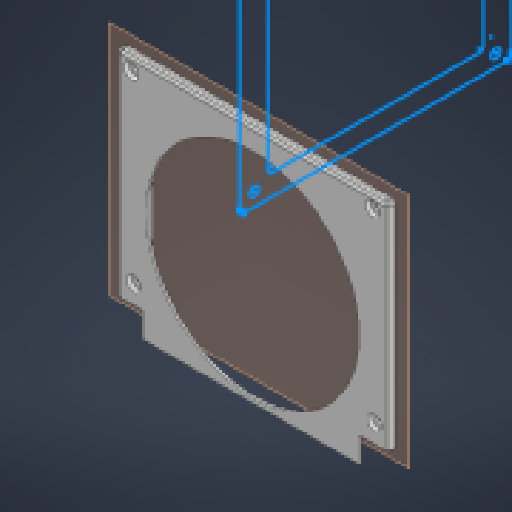
# Autodesk Inventor part: BP_FanCover
Saved by Autodesk Inventor 2026.1 (Build 301233020, 233B)
## iProperties
Created: 2025-09-13
Part Number: BP_FanCover
Material: Generic
Document SubType Name: Modeling
Designer: atrus
Density: 1 g/cm^3
Appearance: Default
Author: atrus
Autodesk Inventor part; units mm, degrees
ref_plane "YZ Plane" through (0, 0, 0) normal (1, 0, 0) x (0, 1, 0)
ref_plane "XZ Plane" through (0, 0, 0) normal (0, 1, 0) x (-1, 0, 0)
ref_plane "XY Plane" through (0, 0, 0) normal (0, 0, 1) x (1, 0, 0)
ref_plane "Work Plane1" through (0, 0, 0) normal (0, 0, 1) x (1, 0, 0)
sketch "Sketch1" plane through (0, 0, 0) normal (0, 0, 1) x (1, 0, 0)
  circle A0 centre (-100.824, -72) radius 2
  circle A1 centre (2.867, -72) radius 2
  circle A2 centre (-101.9061, 6.8071) radius 2
  circle A3 centre (2.0738, 7.3071) radius 2
  spline S0 degree 3 poles (-108.332, 10.6) (-108.332, 10.8603) (-108.2812, 11.1181) (-108.0835, 11.5997) (-107.9386, 11.819) (-107.5727, 12.1898) (-107.3552, 12.3377) (-106.9918, 12.4925) (-106.8631, 12.5326) (-106.5995, 12.5864) (-106.4653, 12.6) (-106.3308, 12.6) knots 0 0 0 0 0.247849 0.247849 0.495777 0.495777 0.743857 0.743857 0.871926 0.871926 1 1 1 1
  line L0 (-108.332, 10.6) -> (-108.332, -80)
  line L1 (-96.066, -80) -> (-108.332, -80)
  line L2 (-96.066, -80) -> (-96.066, 1.6)
  arc A4 (-94.066, 3.6) -> (-96.066, 1.6) centre (-94.066, 1.6) ccw
  line L3 (-94.066, 3.6) -> (-5.266, 3.6)
  arc A5 (-3.266, 1.6) -> (-5.266, 3.6) centre (-5.266, 1.6) ccw
  line L4 (-3.266, -80) -> (-3.266, 1.6)
  line L5 (-3.266, -80) -> (9, -80)
  line L6 (9, 10.6) -> (9, -80)
  spline S1 degree 3 poles (6.9988, 12.6) (7.2595, 12.6) (7.5178, 12.5491) (8.0001, 12.3511) (8.2196, 12.206) (8.5905, 11.8399) (8.7383, 11.6225) (8.8929, 11.2593) (8.9329, 11.1309) (8.9865, 10.868) (9, 10.7342) (9, 10.6) knots 0 0 0 0 0.248262 0.248262 0.49645 0.49645 0.744488 0.744488 0.872247 0.872247 1 1 1 1
  line L7 (-106.3308, 12.6) -> (6.9988, 12.6)
  point P0 (0, 0)
extrude "Extrusion1" add sketch "Sketch1" along normal blind 2 contours A0 | A1 | A2 | A3 | S0 L7 S1 L6 L5 L4 A5 L3 A4 L2 L1 L0
sketch "Sketch2" plane through (0, 0, 2) normal (0, 0, 1) x (1, 0, 0)
  line L0 (9, -80) -> (9, 10.6) projected
  ellipse E0 centre (6.9988, 10.6) end of major axis (8.9999, 10.5798) minor radius 2 (9, 10.6) -> (6.9988, 12.6) ccw projected
  line L1 (6.9988, 12.6) -> (-106.3308, 12.6) projected
  ellipse E1 centre (-106.3308, 10.6) end of major axis (-104.3298, 10.6202) minor radius 2 (-106.3308, 12.6) -> (-108.332, 10.6) ccw projected
  line L2 (-108.332, 10.6) -> (-108.332, -80) projected
  line L3 (8.2, -80) -> (8.2, 10.6)
  line L4 (6.9988, 11.8) -> (-106.3308, 11.8)
  line L5 (-107.532, 10.6) -> (-107.532, -80)
  circle A0 centre (-49.666, -42.9) radius 0.5 projected
  circle A1 centre (-49.666, -42.9) radius 46
  line L6 (8.2, -80) -> (-3.466, -80)
  line L7 (-3.466, -80) -> (-3.466, -90.9)
  line L8 (-3.466, -90.9) -> (-97.166, -90.9)
  line L9 (-97.166, -90.9) -> (-97.166, -80)
  line L10 (-97.166, -80) -> (-107.532, -80)
  line L11 (-97.366, -98.2561) -> (-97.366, -79.6439) construction
  spline S0 degree 5 poles (8.2, 10.6) (8.2001, 10.9773) (8.052, 11.3547) (7.7535, 11.6524) (7.3761, 11.8001) (6.9988, 11.8) knots 0 0 0 0 0 0 1 1 1 1 1 1
  spline S1 degree 5 poles (-106.3308, 11.8) (-106.7081, 11.8001) (-107.0855, 11.6524) (-107.384, 11.3547) (-107.5321, 10.9773) (-107.532, 10.6) knots 0 0 0 0 0 0 1 1 1 1 1 1
  point P0 (0, 0)
  point P1 (-96.066, -80)
  point P2 (-3.266, -80)
  dimension "d2" = 0.8
  dimension "d3" = 92
  dimension "d5" = 0.2
  dimension "d6" = 48
  dimension "d18" = 0.2
  constraints: 16 end point, 5 parallel, 3 perpendicular, 2 point on line, 1 centre point, 1 coincident, 1 horizontal, 8 other
  measures "d2" distance between parallel lines of L0 L3
  measures "d3" diameter of A1
  measures "d5" distance from line of point (-3.266, -80) L7
  measures "d6" distance from line of L8 A0.centre
  measures "d18" distance between parallel lines of L11 L9
extrude "Extrusion2" add sketch "Sketch2" along normal blind 1 contours L6 L7 L8 L9 L10 L5 S1 L4 S0 L3
sketch "Sketch3" plane through (0, 0, 3) normal (0, 0, 1) x (1, 0, 0)
  circle A0 centre (2.0738, 7.3071) radius 2 construction
  circle A1 centre (2.867, -72) radius 2 construction
  circle A2 centre (-100.824, -72) radius 2 construction
  circle A3 centre (-101.9061, 6.8071) radius 2 construction
  point P0 (0, 0)
  constraints: 4 coincident
hole "Hole1" at (2.0738, 7.3071, 3) at (-101.9061, 6.8071, 3) at (-100.824, -72, 3) at (2.867, -72, 3) direction (0, 0, -1) diameter 3.4 end through all counterbore diameter 6.3 counterbore depth 2 clearance for "Flat Head Machine Screw" size "M3" standard "Ansi Metric M Profile"
sketch "Sketch4" plane through (0, 0, 2) normal (0, 0, 1) x (1, 0, 0)
  line L0 (8.2, 10.6) -> (8.2, -80) projected
  line L1 (8.2, -80) -> (9, -80) projected
  line L2 (9, -80) -> (9, 10.6) projected
  ellipse E0 centre (6.9988, 10.6) end of major axis (8.9999, 10.5798) minor radius 2 (9, 10.6) -> (6.9988, 12.6) ccw projected
  line L3 (6.9988, 12.6) -> (-106.3308, 12.6) projected
  ellipse E1 centre (-106.3308, 10.6) end of major axis (-104.3298, 10.6202) minor radius 2 (-106.3308, 12.6) -> (-108.332, 10.6) ccw projected
  line L4 (-108.332, 10.6) -> (-108.332, -80) projected
  line L5 (-108.332, -80) -> (-107.532, -80) projected
  line L6 (-107.532, -80) -> (-107.532, 10.6) projected
  ellipse E2 centre (-106.3308, 10.6) end of major axis (-105.1298, 10.6126) minor radius 1.2 (-106.3308, 11.8) -> (-107.532, 10.6) ccw projected
  line L7 (-106.3308, 11.8) -> (6.9988, 11.8) projected
  ellipse E3 centre (6.9988, 10.6) end of major axis (8.1999, 10.5875) minor radius 1.2 (8.2, 10.6) -> (6.9988, 11.8) ccw projected
  point P0 (0, 0)
  constraints: 4 other
extrude "Extrusion3" add sketch "Sketch4" along normal blind 1
chamfer "Chamfer1" distance 1 angle 45 5 edges at (-49.666, 12.6, 3) (-107.7459, 12.0142, 3) (-108.332, -34.7, 3) (8.4139, 12.0142, 3) (9, -34.7, 3)
body "Solid1"
